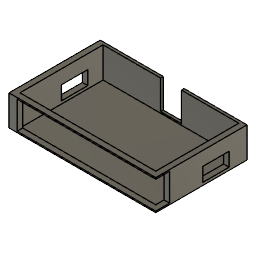
Easyhub-Case (Updated) (Autodesk Fusion 360 archive; units mm, degrees)
design "Case"
part number: 2026-02-02-21-55-55-740
Autodesk Fusion 360 part; units mm, degrees
sketch "Sketch1" plane through (0, 0, 0) normal (0, 0, 1) x (1, 0, 0)
  line L0 (-21.4951, 24.9409) -> (76.5049, 24.9409)
  line L1 (76.5049, 24.9409) -> (76.5049, -35.0591)
  line L2 (76.5049, -35.0591) -> (-21.4951, -35.0591)
  line L3 (-21.4951, -35.0591) -> (-21.4951, 24.9409)
  dimension "d1" = 98
  dimension "d2" = 60
  constraint horizontal L0
  constraint vertical L1
  constraint horizontal L2
  constraint vertical L3
  measures "d1" distance of L0.start L0.end
  measures "d2" distance of L0.start L2.end
extrude "Extrude1" add sketch "Sketch1" along normal blind 2 makes body 1
sketch "Sketch2" plane through (0, 0, 2) normal (0, 0, 1) x (-1, 0, 0)
  line L0 (21.4951, 35.0591) -> (-76.5049, 35.0591)
  line L1 (-76.5049, 35.0591) -> (-76.5049, -24.9409)
  line L2 (-76.5049, -24.9409) -> (21.4951, -24.9409)
  line L3 (21.4951, -24.9409) -> (21.4951, 35.0591)
  line L4 (25.4951, -26.9409) -> (-80.5049, -26.9409)
  line L5 (-80.5049, -26.9409) -> (-80.5049, 39.0591)
  line L6 (-80.5049, 39.0591) -> (25.4951, 39.0591)
  line L7 (25.4951, 39.0591) -> (25.4951, -26.9409)
  dimension "d5" = 106
  dimension "d6" = 66
  dimension "d8" = 4
  dimension "d41" = 2
  constraint horizontal L4
  constraint vertical L5
  constraint horizontal L6
  constraint vertical L7
  measures "d5" distance of L4.start L4.end
  measures "d6" distance of L4.start L6.end
  measures "d8" distance of L3 L7
  measures "d41" distance of L2 L4
extrude "Extrude2" add sketch "Sketch2" along normal blind 42 separate body makes body 2
extrude "Extrude3" cut 1 faces at (43.8383, -37.7258, 44) along direction (0, 0, -1) blind 20 on bodies 2 bodies 2
sketch "Sketch3" plane through (0, -39.0591, 0) normal (0, -1, 0) x (1, 0, 0)
  line L0 (80.5049, 24) -> (-25.4951, 24)
  line L1 (-25.4951, 24) -> (-25.4951, 2)
  line L2 (-25.4951, 2) -> (80.5049, 2)
  line L3 (80.5049, 2) -> (80.5049, 24)
  line L4 (-19.4951, 3) -> (86.5049, 3)
  line L5 (86.5049, 3) -> (86.5049, 23)
  line L6 (86.5049, 23) -> (-19.4951, 23)
  line L7 (-19.4951, 23) -> (-19.4951, 3)
  dimension "d13" = 106
  dimension "d14" = 20
  dimension "d15" = 1
  dimension "d16" = 6
  constraint horizontal L4
  constraint vertical L5
  constraint horizontal L6
  constraint vertical L7
  measures "d13" distance of L4.start L4.end
  measures "d14" distance of L4.start L6.end
  measures "d15" distance of L2 L4
  measures "d16" distance of L1 L7
extrude "Extrude4" cut sketch "Sketch3" against normal blind 10 contours L3 L4 L5 L6 | L3 L4 L6 L7 bodies 2
sketch "Sketch4" plane through (80.5049, 0, 0) normal (1, 0, 0) x (0, 1, 0)
  line L0 (26.9409, 24) -> (-39.0591, 24)
  line L1 (-39.0591, 3) -> (-39.0591, 2)
  line L2 (-39.0591, 2) -> (26.9409, 2)
  line L3 (26.9409, 2) -> (26.9409, 24)
  line L4 (-5.0591, 14) -> (13.9409, 14)
  line L5 (13.9409, 14) -> (13.9409, 4)
  line L6 (13.9409, 4) -> (-5.0591, 4)
  line L7 (-5.0591, 4) -> (-5.0591, 14)
  line L8 (-29.0591, 3) -> (-39.0591, 3)
  line L9 (-39.0591, 24) -> (-39.0591, 23)
  line L10 (-39.0591, 23) -> (-29.0591, 23)
  line L11 (-29.0591, 23) -> (-29.0591, 3)
  dimension "d28" = 19
  dimension "d29" = 10
  dimension "d30" = 13
  dimension "d33" = 2
  constraint horizontal L4
  constraint vertical L5
  constraint horizontal L6
  constraint vertical L7
  measures "d28" distance of L4.start L4.end
  measures "d29" distance of L4.start L6.end
  measures "d30" distance of L3 L5
  measures "d33" distance of L2 L6
extrude "Extrude5" cut sketch "Sketch4" against normal blind 120 contours L4 L5 L6 L7 bodies 2
sketch "Sketch5" plane through (0, 26.9409, 0) normal (0, 1, 0) x (-1, 0, 0)
  line L0 (25.4951, 24) -> (-80.5049, 24)
  line L1 (-80.5049, 24) -> (-80.5049, 2)
  line L2 (-80.5049, 2) -> (25.4951, 2)
  line L3 (25.4951, 2) -> (25.4951, 24)
  line L4 (-35.0049, 83) -> (-20.0049, 83)
  line L5 (-20.0049, 83) -> (-20.0049, 3)
  line L6 (-20.0049, 3) -> (-35.0049, 3)
  line L7 (-35.0049, 3) -> (-35.0049, 83)
  dimension "d34" = 15
  dimension "d35" = 80
  dimension "d36" = 1
  dimension "d37" = 45.5
  constraint horizontal L4
  constraint vertical L5
  constraint horizontal L6
  constraint vertical L7
  measures "d34" distance of L4.start L4.end
  measures "d35" distance of L4.start L6.end
  measures "d36" distance of L2 L6
  measures "d37" distance of L3 L5
extrude "Extrude6" cut sketch "Sketch5" against normal blind 10 contours L0 L5 L6 L7 | L0 L4 L5 L7 bodies 2
